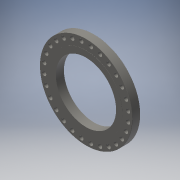
# Autodesk Inventor part: A1-19010-100-01 30in CL300 RFBL flange - raw
Saved by Autodesk Inventor 2017 SP1 (Build 210196100, 196)
## iProperties
Created: 2014-07-18
Part Number: A1-19010-100-01 30in CL300 RFBL flange - raw
Material: A105N
Document SubType Name: Modeling
Designer: Graeme_Van_Dongen
Density: 7.85 g/cm^3
Appearance: Steel - Cast
Mass: 362189 g
Surface Area: 18963.9 cm^2
Volume: 46138.7 cm^3
Description: Ø30" CLASS 300 RFBL FLANGE, A105N, ASME B16.47 Ser.A - CUSTOM
od: 43.000 in
Author: Graeme_Van_Dongen
Autodesk Inventor part; units mm, degrees
ref_plane "YZ Plane" through (0, 0, 0) normal (1, 0, 0) x (0, 1, 0)
ref_plane "XY Plane" through (0, 0, 0) normal (0, 0, 1) x (1, 0, 0)
sketch "Sketch1" plane through (0, 0, 0) normal (0, 0, 1) x (1, 0, 0)
  circle A0 centre (0, 0) radius 546.1
  dimension "d0" = 1092.2
  constraints: 1 centre point, 1 coincident
  measures "d0" diameter of A0
extrude "Extrusion: OD" add sketch "Sketch1" along normal blind 93.6625
sketch "Sketch2" plane through (0, 0, 93.6625) normal (0, 0, 1) x (1, 0, 0)
  circle A0 centre (0, 0) radius 428.625
  dimension "d3" = 857.25
  constraints: 1 centre point, 1 coincident
  measures "d3" diameter of A0
extrude "Extrusion: RF" add sketch "Sketch2" along normal blind 1.5875
sketch "Sketch3" plane through (0, 0, 95.25) normal (0, 0, 1) x (1, 0, 0)
  circle A0 centre (0, -6.35) radius 381
  point P0 (0, 0)
  dimension "d6" = 762
  dimension "d32" = 6.35
  constraints: 1 centre point, 1 vertical alignment
  measures "d6" diameter of A0
  measures "d32" distance of point (0, 0) A0.centre
extrude "Extrusion: ID Large" [suppressed]
sketch "Sketch4" plane through (0, 0, 95.25) normal (0, 0, 1) x (1, 0, 0)
  circle A0 centre (0, 0) radius 355.6
  circle A1 centre (0, 0) radius 428.625 projected
  dimension "d9" = 711.2
  constraints: 1 centre point, 1 coincident
  measures "d9" diameter of A0
extrude "Extrusion: ID Small" cut sketch "Sketch4" along normal through all both and the other way through all contours A0
sketch "Sketch5" plane through (0, 0, 95.25) normal (0, 0, 1) x (1, 0, 0)
  line L0 (-495.3407, -55.8115) -> (495.3407, 55.8115)
  line L1 (-495.3407, -55.8115) -> (501.6093, -55.8115) construction
  point P0 (0, 0)
  point P1 (0, 0)
  dimension "d12" = 996.95
  dimension "d13" = 6.429
  constraints: 4 end point, 2 coincident, 1 equal length, 1 horizontal, 1 midpoint
  measures "d12" distance of L0.start L0.end
  measures "d13" angle of L1 L0
hole "Hole: Bolt" at (495.3407, 55.8115, 95.25) direction (0, 0, -1) diameter 47.625 end through all
chamfer "Chamfer: Bolt hole" distance 1.5875 angle 45 2 edges at (495.3407, 79.624, 93.6625) (495.3407, 79.624, 0)
pattern_circular "Circular Pattern: Bolt hole" count 28 over 360 about axis through (0, 0, -10) along (0, 0, 1) of "Hole: Bolt", "Chamfer: Bolt hole"
chamfer "Chamfer: OD" distance 1.5875 angle 45 2 edges at (-546.1, 0, 93.6625) (-546.1, 0, 0)
chamfer "Chamfer2" [suppressed]
fillet "Fillet2" [suppressed]
ref_plane "Work Plane1" through (0, 546.1, 0) normal (0, 1, 0) x (-1, 0, 0)
sketch "Sketch6" plane through (0, 546.1, 0) normal (0, 1, 0) x (-1, 0, 0)
  point P0 (0, 0)
  point P1 (0, 47.625)
  dimension "d36" = 47.625
  constraints: 1 vertical alignment
  measures "d36" distance of point (0, 0) point (0, 47.625)
hole "Hole2" [suppressed]
pattern_circular "Circular Pattern2" [suppressed]
equation "\"d0\" = od"
equation "\"d1\" = thk - rf"
equation "\"d3\" = od_rf"
equation "\"d4\" = rf"
equation "\"d6\" = id_large"
equation "\"d9\" = id_large - 2 * r_diff_id"
equation "\"d36\" = 0.5 * d4 + 0.5 * d1"
equation "\"od\" = 1092.2"
equation "\"thk\" = 95.25"
equation "\"rf\" = 1.5875"
equation "\"od_rf\" = 857.25"
equation "\"id_large\" = 762"
equation "\"r_diff_id\" = 25.4"
body "Solid1"
